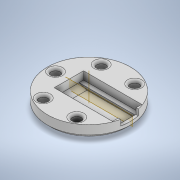
# Autodesk Inventor part: hmmb
Saved by Autodesk Inventor 2021 (Build 250183000, 183)
## iProperties
Created: 2020-07-09
Part Number: hmmb
Material: Generic
Document SubType Name: Modeling
Designer: andre
Density: 1 g/cm^3
Appearance: Default
Author: andre
## iProperties of the stored document _3DPrint.ipt
Created: 2020-07-09
Part Number: _3DPrint
Material: Generic
Document SubType Name: Modeling
Designer: andre
Density: 1 g/cm^3
Appearance: Default
Author: andre
Autodesk Inventor part; units mm, degrees
note: some values were not read from the file. Chosen so that the rebuilt part matches the saved one: pattern direction of "Circular Pattern2".
ref_plane "YZ Plane" through (0, 0, 0) normal (1, 0, 0) x (0, 1, 0)
ref_plane "XZ Plane" through (0, 0, 0) normal (0, 1, 0) x (-1, 0, 0)
ref_plane "XY Plane" through (0, 0, 0) normal (0, 0, 1) x (1, 0, 0)
sketch "Sketch1" plane through (0, 0, 0) normal (0, 1, 0) x (-1, 0, 0)
  circle A0 centre (0, 0) radius 26
  dimension "d0" = 52
  constraints: 1 centre point
  measures "d0" diameter of A0
extrude "Extrusion1" add sketch "Sketch1" along normal blind 7.6
chamfer "Chamfer2" distance 2 angle 45 1 edges at (26, 0, 0)
sketch "Sketch2" plane through (0, 7.6, 0) normal (0, 1, 0) x (1, 0, 0)
  line L0 (-12.6, -9.19) -> (23.96, -9.19)
  line L1 (23.96, -9.19) -> (23.96, 9.19)
  line L2 (23.96, 9.19) -> (-12.6, 9.19)
  line L3 (-12.6, 9.19) -> (-12.6, -9.19)
  point P0 (0, 0)
  dimension "d5" = 36.56
  dimension "d6" = 18.38
  dimension "d7" = 9.19
  dimension "d8" = 12.6
  constraints: 8 end point, 2 parallel, 1 horizontal, 1 perpendicular
  measures "d5" distance of L2.end L1.end
  measures "d6" distance of L1.end L0.end
  measures "d7" distance from line of point (0, 0) L2
  measures "d8" distance from line of point (0, 0) L3
extrude "Extrusion2" cut sketch "Sketch2" against normal blind 5
sketch "Sketch3" plane through (23.96, 7.6, -9.19) normal (-1, 0, 0) x (0, 0, 1)
  line L0 (3.6, 0) -> (14.78, 0)
  line L1 (14.78, 0) -> (14.78, -3.6)
  line L2 (14.78, -3.6) -> (3.6, -3.6)
  line L3 (3.6, -3.6) -> (3.6, 0)
  line L4 (0, 0) -> (18.38, 0) projected
  line L5 (0, -5) -> (18.38, -5) projected
  line L6 (0, 0) -> (0, -5) projected
  line L7 (18.38, 0) -> (18.38, -5) projected
  point P0 (9.19, -7.6)
  dimension "d11" = 0
  dimension "d14" = 3.6
  dimension "d44" = 3.6
  dimension "d47" = 1.4
  constraints: 8 end point, 2 parallel, 1 horizontal, 1 perpendicular
  measures "d11" distance between parallel lines of L4 L0
  measures "d14" distance between parallel lines of L7 L1
  measures "d44" distance between parallel lines of L6 L3
  measures "d47" distance between parallel lines of L5 L2
extrude "Extrusion3" cut sketch "Sketch3" against normal through all contours L0 L1 L2 L3
ref_plane "Work Plane1" through (-12.6, 7.6, 0) normal (0, 0, 1) x (1, 0, 0)
sketch "Sketch7" plane through (0, 2.6, 0) normal (0, 1, 0) x (1, 0, 0)
  line L0 (-12.6, 6.35) -> (22.96, 6.35)
  line L1 (22.96, 6.35) -> (22.96, -6.35)
  line L2 (22.96, -6.35) -> (-12.6, -6.35)
  line L3 (-12.6, -6.35) -> (-12.6, 6.35)
  line L4 (36.4, 0) -> (-36.4, 0) projected
  line L5 (-12.6, -9.19) -> (-12.6, 9.19) projected
  point P0 (0, 0)
  dimension "d28" = 12.7
  dimension "d29" = 35.56
  dimension "d30" = 6.35
  dimension "d31" = 0
  constraints: 8 end point, 2 parallel, 1 horizontal, 1 perpendicular
  measures "d28" distance of L0.end L1.end
  measures "d29" distance between parallel lines of L1 L3
  measures "d30" distance between parallel lines of L4 L0
  measures "d31" distance between parallel lines of L5 L3
extrude "Extrusion5" cut sketch "Sketch7" against normal blind 1.6
sketch "Sketch4" plane through (0, 7.6, 0) normal (0, 1, 0) x (1, 0, 0)
  circle A0 centre (-21, 0) radius 2.8
  arc A1 (25.392, 5.59) -> (25.392, -5.59) centre (0, 0) ccw projected
  point P0 (24.6995, 8.12)
  point P1 (24.6995, -8.12)
  dimension "d17" = 5.6
  dimension "d23" = 21
  constraints: 1 centre point
  measures "d17" diameter of A0
  measures "d23" distance of A0.centre A1.centre
extrude "Extrusion4" cut sketch "Sketch4" against normal blind 5.2
fillet "Fillet4" radius 1.6 1 edges at (-23.8, 7.6, 0)
pattern_circular "Circular Pattern2" count 5 over 240 about axis through (0, 7.6, 0) along (0, 1, 0) of "Extrusion4", "Fillet4" both ways yes
chamfer "Chamfer3" distance 1.5 distance2 5 1 edges at (-12.6, 1, 0) measured on face at (-12.6, 5.9333, -2.1167)
equation "\"d7\" = 0.5 * d6"
equation "\"d44\" = d14"
equation "\"d30\" = 0.5 * d28"
equation "\"d24\" = 0.5 * d6"
body "Solid1"
